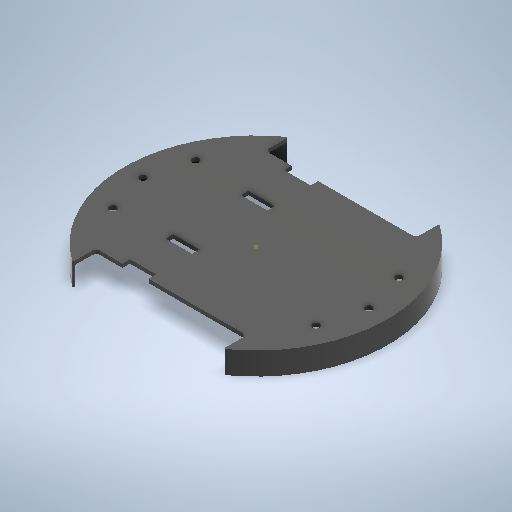
# Autodesk Inventor part: base 1
Saved by Autodesk Inventor 2025.1 (Build 291241000, 241)
## iProperties
Created: 2024-09-05
Part Number: base 1
Material: Plástico PC/ABS
Document SubType Name: Modeling
Designer: Célio
Density: 1.1 g/cm^3
Appearance: Suave - Preto
Author: Célio
Autodesk Inventor part; units mm, degrees
ref_plane "YZ Plane" through (0, 0, 0) normal (1, 0, 0) x (0, 1, 0)
ref_plane "XZ Plane" through (0, 0, 0) normal (0, 1, 0) x (-1, 0, 0)
ref_plane "XY Plane" through (0, 0, 0) normal (0, 0, 1) x (1, 0, 0)
sketch "Esboço1" plane through (0, 0, 0) normal (0, 1, 0) x (-1, 0, 0)
  line L0 (-40, 47) -> (-40, 56.4801)
  line L1 (40, 56.4801) -> (40, 47)
  line L2 (-40, -47) -> (-40, -56.4801)
  line L3 (40, -56.4801) -> (40, -47)
  arc A0 (-40.7914, 56.8864) -> (-40.7914, -56.8864) centre (0, 0) ccw
  arc A1 (40.7914, -56.8864) -> (40.7914, 56.8864) centre (0, 0) ccw
  line L4 (12, 45) -> (12, 41)
  line L5 (12, -45) -> (12, -43)
  line L6 (26, -43) -> (26, -45)
  line L7 (0, 45) -> (12, 45)
  line L8 (26, 45) -> (38, 45)
  line L9 (38, 45) -> (26, 45)
  line L10 (12, 45) -> (-38, 45)
  line L11 (38, -45) -> (26, -45)
  line L12 (12, -45) -> (-38, -45)
  line L13 (0, -45) -> (12, -45)
  line L14 (26, -45) -> (38, -45)
  line L15 (26, 22) -> (12, 22)
  line L16 (12, 22) -> (12, 20)
  line L17 (26, 19.2) -> (26, 22)
  line L18 (26, -22) -> (12, -22)
  line L19 (12, -22) -> (12, -18)
  line L20 (12, -18) -> (26, -18)
  line L21 (26, -18) -> (26, -22)
  arc A2 (40, -47) -> (38, -45) centre (38, -47) ccw
  arc A3 (-38, -45) -> (-40, -47) centre (-38, -47) ccw
  arc A4 (-40, 47) -> (-38, 45) centre (-38, 47) ccw
  arc A5 (38, 45) -> (40, 47) centre (38, 47) ccw
  circle A6 centre (54, 22) radius 2
  circle A7 centre (54, -22) radius 2
  circle A8 centre (-54, -22) radius 2
  circle A9 centre (-54, 22) radius 2
  arc A10 (40.7914, 56.8864) -> (40, 56.4801) centre (40.5, 56.4801) ccw
  arc A11 (-40, 56.4801) -> (-40.7914, 56.8864) centre (-40.5, 56.4801) ccw
  arc A12 (-40.7914, -56.8864) -> (-40, -56.4801) centre (-40.5, -56.4801) ccw
  arc A13 (40, -56.4801) -> (40.7914, -56.8864) centre (40.5, -56.4801) ccw
  circle A14 centre (60, 0) radius 2
  circle A15 centre (-60, 0) radius 2
  line L22 (26, 22) -> (12, 22)
  line L23 (12, 22) -> (12, 18)
  line L24 (12, 18) -> (26, 18)
  line L25 (26, 18) -> (26, 22)
  line L26 (12, 41) -> (26, 41)
  line L27 (26, 41) -> (26, 45)
  line L28 (12, 44.2) -> (12, 41)
  line L29 (26, -45) -> (26, -41)
  line L30 (26, -41) -> (12, -41)
  line L31 (12, -41) -> (12, -45)
  point P0 (-40, 57.4456)
  point P1 (40, 57.4456)
  point P2 (-40, -57.4456)
  point P3 (40, -57.4456)
  dimension "d69" = 0.5
  dimension "d76" = 4
  dimension "d77" = 4
  dimension "d80" = 4
  dimension "d81" = 4
  dimension "d83" = 19
  dimension "d84" = 14
  dimension "d86" = 19
  dimension "d87" = 4
  constraints: 64 end point, 24 point on circle, 16 centre point, 16 tangent, 12 horizontal, 10 parallel, 8 perpendicular, 6 equal radius, 4 point on line
  measures "d69" radius of A10
  measures "d76" diameter of A14
  measures "d77" diameter of A15
  measures "d80" distance of L4.start L4.end
  measures "d81" distance of L22.end L23.end
  measures "d83" distance between parallel lines of L15 L26
  measures "d84" distance of L23.end L24.end
  measures "d86" distance between parallel lines of L18 L30
  measures "d87" distance of L18.end L19.end
extrude "Extrusão1" add sketch "Esboço1" along normal blind 2
sketch "Esboço2" plane through (0, 0, 0) normal (0, -1, 0) x (1, 0, 0)
  point P0 (0, 0)
sketch "Esboço3" plane through (0, 0, 0) normal (0, -1, 0) x (1, 0, 0)
  line L0 (40, 47) -> (40, 56.4801) projected
  line L1 (40, 56.2228) -> (40, 56.4801)
  line L2 (-40, 56.2228) -> (-40, 56.4801)
  line L3 (-40, -56.2228) -> (-40, -56.4801)
  line L4 (40, -56.2228) -> (40, -56.4801)
  arc A0 (40, -56.2228) -> (40, 56.2228) centre (0, 0) ccw
  arc A1 (-40, 56.2228) -> (-40, -56.2228) centre (0, 0) ccw
  arc A2 (40.7914, -56.8864) -> (40.7914, 56.8864) centre (0, 0) ccw
  arc A3 (-40.7914, 56.8864) -> (-40.7914, -56.8864) centre (0, 0) ccw
  arc A4 (40.7914, 56.8864) -> (40, 56.4801) centre (40.5, 56.4801) ccw
  arc A5 (-40, 56.4801) -> (-40.7914, 56.8864) centre (-40.5, 56.4801) ccw
  arc A6 (-40.7914, -56.8864) -> (-40, -56.4801) centre (-40.5, -56.4801) ccw
  arc A7 (40, -56.4801) -> (40.7914, -56.8864) centre (40.5, -56.4801) ccw
  point P0 (40, 57.4456)
  point P1 (-40, 57.4456)
  point P2 (-40, -57.4456)
  point P3 (40, -57.4456)
  point P4 (40, 56.4801)
  dimension "d71" = 0.5
  constraints: 20 point on circle, 8 centre point, 8 end point, 8 point on line, 8 tangent, 3 equal radius, 2 coincident, 1 collinear, 1 parallel
  measures "d71" radius of A4
extrude "Extrusão2" add sketch "Esboço3" along normal blind 10
